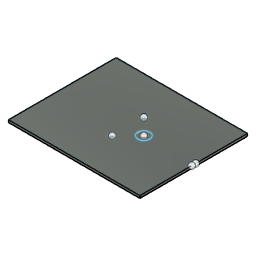
acces3c (Autodesk Fusion 360 design; units mm, degrees)
Autodesk Fusion 360 part; units mm, degrees
box "BoxPrimitive1" add length 136 width 166 height 3 placed x (0, -1, 0) y (1, 0, 0) z (0, 0, 1) at (-30, 40, 0)
move_body "Move1" bodies 1 to x (1, 0, 0) y (0, 1, 0) z (0, 0, 1) at (-59.3373, 23.0424, 23.0424)
move_body "Move2" bodies 1 to x (1, 0, 0) y (0, 1, 0) z (0, 0, 1) at (6.3373, 4.9576, -26.0424)
move_body "Move3" bodies 1 to x (1, 0, 0) y (0, 1, 0) z (0, 0, 1) at (0, 0, 3)
sketch "Sketch4" plane through (0, 0, 3) normal (0, 0, 1) x (-1, 0, 0)
  line L0 (83, 68) -> (-83, 68)
  line L1 (-83, 68) -> (-83, -68)
  line L2 (-83, -68) -> (83, -68)
  line L3 (83, -68) -> (83, 68)
  line L4 (1, -18.5) -> (-1, -18.5)
  line L5 (-1, -18.5) -> (-1, -21.5)
  line L6 (-1, -21.5) -> (1, -21.5)
  line L7 (1, -21.5) -> (1, -18.5)
  line L8 (-1, 18.5) -> (1, 18.5)
  line L9 (1, 18.5) -> (1, 21.5)
  line L10 (1, 21.5) -> (-1, 21.5)
  line L11 (-1, 21.5) -> (-1, 18.5)
  circle A0 centre (-20, 0) radius 7.5
  line L12 (-82, -2.5) -> (-83, -2.5)
  line L13 (-83, 2.5) -> (-82, 2.5)
  line L14 (-82, 2.5) -> (-82, -2.5)
  point P0 (0, -20)
  point P1 (0, 20)
  dimension "d14" = 2
  dimension "d15" = 3
  dimension "d16" = 2
  dimension "d17" = 3
  dimension "d26" = 15
  dimension "d27" = 5
  constraint horizontal L4
  constraint perpendicular L4 L5
  constraint parallel L4 L6
  constraint parallel L5 L7
  constraint horizontal L8
  constraint perpendicular L8 L9
  constraint parallel L8 L10
  constraint parallel L9 L11
  constraint horizontal L12
  constraint horizontal L13
  constraint vertical L14
  measures "d14" distance of L5.end L6.end
  measures "d15" distance of L4.end L5.end
  measures "d16" distance of L9.end L10.end
  measures "d17" distance of L8.end L9.end
  measures "d26" diameter of A0
  measures "d27" distance of L12.start L13.end
extrude "Extrude1" cut sketch "Sketch4" against normal blind 5 contours L4 L5 L6 L7 | L8 L9 L10 L11
